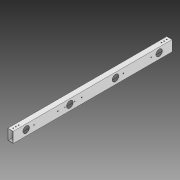
# Autodesk Inventor part: VersaChassis Drive Rail Template
Saved by Autodesk Inventor 2022 (Build 260153000, 153)
## iProperties
Created: 2021-12-11
Part Number: VersaChassis Drive Rail Template
Material: Aluminum
Document SubType Name: Modeling
Designer: Max Boord
Density: 2.7 g/cm^3
Appearance: Satin
Author: Max Boord
Autodesk Inventor part; units mm, degrees
ref_plane "YZ Plane" through (0, 0, 0) normal (1, 0, 0) x (0, 1, 0)
ref_plane "XZ Plane" through (0, 0, 0) normal (0, 1, 0) x (-1, 0, 0)
ref_plane "XY Plane" through (0, 0, 0) normal (0, 0, 1) x (1, 0, 0)
sketch "Sketch1" plane through (0, 0, 0) normal (1, 0, 0) x (0, 1, 0)
  line L0 (25.4, -381) -> (-25.4, -381)
  line L1 (-25.4, -381) -> (-25.4, 381)
  line L2 (-25.4, 381) -> (25.4, 381)
  line L3 (25.4, 381) -> (25.4, -381)
  line L4 (25.4, -381) -> (-25.4, 381) construction
  line L5 (-25.4, -381) -> (25.4, 381) construction
  circle A0 centre (1.5875, -319.0875) radius 15.875
  line L6 (0, -381) -> (0, -205.8364) construction
  circle A1 centre (1.5875, -280.9875) radius 2.4892
  circle A2 centre (1.5875, -280.9875) radius 5.2705
  circle A3 centre (-1.5875, 0) radius 15.875
  line L7 (0, 0) -> (48.0139, 0) construction
  circle A4 centre (1.5875, 319.0875) radius 15.875
  circle A5 centre (1.5875, 280.9875) radius 2.4892
  circle A6 centre (1.5875, 280.9875) radius 5.2705
  circle A7 centre (1.5875, -319.0875) radius 76.2 construction
  circle A8 centre (-1.5875, 0) radius 76.2 construction
  circle A9 centre (1.5875, 319.0875) radius 76.2 construction
  circle A10 centre (-1.5875, -23.8125) radius 2.0193
  circle A11 centre (19.0347, -11.9063) radius 2.0193
  circle A12 centre (19.0347, 11.9062) radius 2.0193
  circle A13 centre (-1.5875, 23.8125) radius 2.0193
  circle A14 centre (-22.2097, 11.9062) radius 2.0193 construction
  circle A15 centre (-22.2097, -11.9063) radius 2.0193 construction
  circle A16 centre (-1.5875, -57.15) radius 2.4892
  circle A17 centre (-1.5875, -57.15) radius 5.2705
  circle A18 centre (-1.5875, 57.15) radius 2.4892
  circle A19 centre (-1.5875, 57.15) radius 5.2705
  circle A20 centre (1.5875, -109.5375) radius 15.875
  circle A21 centre (1.5875, -147.6375) radius 2.4892
  circle A22 centre (1.5875, -147.6375) radius 5.2705
  line L8 (1.5875, 280.9875) -> (1.5875, 319.0875) construction
  line L9 (1.5875, -109.5375) -> (1.5875, -147.6375) construction
  circle A23 centre (1.5875, 85.725) radius 2.0193
  circle A24 centre (1.5875, 52.3875) radius 2.4892
  circle A25 centre (1.5875, 52.3875) radius 5.2705
  circle A26 centre (1.5875, 166.6875) radius 2.4892
  circle A27 centre (1.5875, 166.6875) radius 5.2705
  circle A28 centre (1.5875, 133.35) radius 2.0193
  line L10 (1.5875, 133.35) -> (1.5875, 85.725) construction
  line L11 (-1.5875, 23.8125) -> (-1.5875, -23.8125) construction
  line L12 (1.5875, 166.6875) -> (1.5875, 52.3875) construction
  line L13 (-1.5875, 57.15) -> (-1.5875, -57.15) construction
  circle A29 centre (1.5875, 109.5375) radius 15.875
  line L14 (25.4, 381) -> (-25.4, 381) construction
  line L15 (-25.4, 381) -> (-25.4, 406.4) construction
  line L16 (-25.4, 406.4) -> (25.4, 406.4) construction
  line L17 (25.4, 406.4) -> (25.4, 381) construction
  line L18 (25.4, 404.8125) -> (-25.4, 404.8125) construction
  line L19 (25.4, 401.6375) -> (-25.4, 401.6375) construction
  point P0 (0, 0)
  point P1 (1.5875, 1.5875)
  point P2 (1.5875, -19.5792)
  point P3 (3.2385, -19.5792)
  point P4 (1.5875, -19.5792)
  dimension "d0" = 762
  dimension "d1" = 50.8
  dimension "d2" = 31.75
  dimension "d4" = 10.541
  dimension "d5" = 4.9784
  dimension "d6" = 1.5875
  dimension "d7" = 1.5875
  dimension "d8" = 38.1
  dimension "d9" = 319.0875
  dimension "d10" = 152.4
  dimension "d13" = 4.0386
  dimension "d16" = 360
  dimension "d18" = 4.9784
  dimension "d19" = 10.541
  dimension "d20" = 114.3
  dimension "d21" = 47.625
  dimension "d22" = 3.1903
  dimension "d26" = 4.0386
  dimension "d28" = 4.9784
  dimension "d29" = 10.541
  dimension "d33" = 360
  dimension "d35" = 219.075
  dimension "d36" = 209.55
  dimension "d58" = 25.4
  dimension "d59" = 1.5875
  dimension "d60" = 3.175
  constraints: 40 end point, 30 centre point, 7 equal radius, 7 vertical, 7 vertical alignment, 6 coincident, 5 parallel, 4 midpoint, 4 symmetric about line, 3 equal length, 3 horizontal, 3 perpendicular, 2 horizontal alignment, 2 point on line, 29 other
  measures "d0" distance of L2.end L0.start
  measures "d1" distance between parallel lines of L1 L3
  measures "d2" diameter of A0
  measures "d4" diameter of A2
  measures "d5" diameter of A1
  measures "d6" distance from line of L6 A0.centre
  measures "d7" distance from line of L6 A3.centre
  measures "d8" distance of A1.centre A0.centre
  measures "d9" vertical distance of A4.centre point (0, 0)
  measures "d10" diameter of A9
  measures "d13" diameter of A10
  measures "d18" diameter of A16
  measures "d19" diameter of A17
  measures "d20" distance of L13.end L13.start
  measures "d21" distance of A15.centre A12.centre
  measures "d22" distance from line of L1 A14.centre
  measures "d26" diameter of A23
  measures "d28" diameter of A24
  measures "d29" diameter of A25
  measures "d35" distance of point (1.587, 109.537) A20.centre
  measures "d36" distance of A4.centre point (1.587, 109.537)
  measures "d58" distance of L1.end L15.end
  measures "d59" distance between parallel lines of L16 L18
  measures "d60" distance between parallel lines of L18 L19
extrude "Extrusion1" add sketch "Sketch1" along normal mid plane 25.4 contours L0 L1 L2 L3 | A2 | A3 | A6 | A10 | A11 | A12 | A13 | A16 | A17 | A18 A25 | A18 A25 A19 A24 | A25 A18 | A18 A25 A19 | A25 A19 A24 | A22 | A27
sketch "Sketch2" plane through (-12.7, -25.4, -381) normal (0, 0, -1) x (-1, 0, 0)
  line L0 (0, 50.8) -> (-25.4, 50.8) projected
  line L1 (-25.4, 0) -> (-25.4, 50.8) projected
  line L2 (0, 50.8) -> (0, 0) projected
  line L3 (-23.8125, 49.2125) -> (-1.5875, 49.2125)
  line L4 (-1.5875, 49.2125) -> (-1.5875, 1.5875)
  line L5 (-1.5875, 1.5875) -> (-23.8125, 1.5875)
  line L6 (-23.8125, 1.5875) -> (-23.8125, 49.2125)
  line L7 (0, 0) -> (-25.4, 0) projected
  point P0 (-12.7, 25.4)
  dimension "d23" = 1.5875
  constraints: 8 end point, 1 other
  measures "d23" distance between parallel lines of L0 L3
extrude "Extrusion2" cut sketch "Sketch2" against normal through all contours L3 L4 L5 L6
sketch "Sketch3" plane through (-12.7, 25.4, 381) normal (0, 1, 0) x (1, 0, 0)
  line L0 (0, 762) -> (25.4, 762) projected
  line L1 (0, 762) -> (25.4, 762) projected
  line L2 (12.7, 762) -> (12.7, 749.3)
  circle A0 centre (12.7, 749.3) radius 2.4892
  circle A1 centre (12.7, 736.6) radius 2.4892
  circle A2 centre (12.7, 723.9) radius 2.4892
  line L3 (12.7, 381) -> (42.3415, 381) construction
  circle A3 centre (12.7, 12.7) radius 2.4892
  circle A4 centre (12.7, 25.4) radius 2.4892
  circle A5 centre (12.7, 38.1) radius 2.4892
  dimension "d37" = 12.7
  dimension "d38" = 4.9784
  dimension "d41" = 12.7
  constraints: 6 centre point, 4 end point, 4 symmetric about line, 2 coincident, 2 vertical, 1 horizontal, 1 midpoint, 7 other
  measures "d37" distance of L2.start L2.end
  measures "d38" diameter of A0
  measures "d41" distance of A0.centre A1.centre
extrude "Extrusion3" cut sketch "Sketch3" against normal through all
sketch "Sketch4" plane through (-12.7, 0, 0) normal (-1, 0, 0) x (0, 0, 1)
  circle A0 centre (280.9875, 1.5875) radius 2.4892 projected
  circle A1 centre (-280.9875, 1.5875) radius 2.4892 projected
  circle A2 centre (52.3875, 1.5875) radius 2.4892 projected
  circle A3 centre (166.6875, 1.5875) radius 2.4892 projected
  circle A4 centre (-147.6375, 1.5875) radius 2.4892 projected
  point P0 (0, 0)
  point P1 (57.15, -1.5875)
  constraints: 5 coincident
hole "Hole1" at (-12.7, 1.5875, 280.9875) at (-12.7, 1.5875, 52.3875) at (-12.7, 1.5875, 166.6875) at (-12.7, 1.5875, -280.9875) at (-12.7, 1.5875, -147.6375) direction (1, 0, 0) diameter 4.9784 depth 25.4 tip angle 118 counterbore diameter 10.541 counterbore depth 4.826 clearance for "Socket Head Cap Screw" size "#10" standard "Ansi Unified Screw Threads"
equation "\"d7\" = d6"
body "Solid1"
